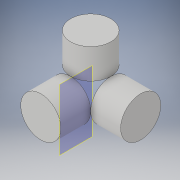
# Autodesk Inventor part: 3-way 90 1 Inch
Saved by Autodesk Inventor 2018 (Build 220112000, 112)
## iProperties
Created: 2018-01-18
Part Number: 3-way 90 1 Inch
Material: Generic
Document SubType Name: Modeling
Designer: owner
Density: 1 g/cm^3
Appearance: Default
Author: owner
Autodesk Inventor part; units mm, degrees
ref_plane "YZ Plane" through (0, 0, 0) normal (1, 0, 0) x (0, 1, 0)
ref_plane "XZ Plane" through (0, 0, 0) normal (0, 1, 0) x (-1, 0, 0)
ref_plane "XY Plane" through (0, 0, 0) normal (0, 0, 1) x (1, 0, 0)
sketch "Sketch11" plane through (0, 0, 0) normal (0, 0, 1) x (1, 0, 0)
  circle A0 centre (0, 0) radius 20.3835
  dimension "d30" = 40.767
  constraints: 1 centre point, 1 coincident
  measures "d30" diameter of A0
extrude "Extrusion7" add sketch "Sketch11" against normal blind 30.4292
sketch "Sketch12" plane through (0, 0, -30.4292) normal (0, 0, -1) x (-1, 0, 0)
  circle A0 centre (0, 0) radius 20.3835 projected
  line L0 (-20.3835, 0) -> (-20.3835, 36.5355)
  line L1 (0, 20.3835) -> (-34.8493, 20.3835)
  constraints: 4 end point, 2 point on circle, 2 tangent, 1 horizontal, 1 vertical
ref_plane "Work Plane4" through (20.3835, 0, -30.4292) normal (-1, 0, 0) x (0, 1, 0)
sketch "Sketch13" plane through (20.3835, 0, -30.4292) normal (-1, 0, 0) x (0, 1, 0)
  line L0 (0, -30.4292) -> (0, 20.3708)
  circle A0 centre (0, 20.3708) radius 20.3835
  line L1 (20.3835, 0) -> (-20.3835, 0) projected
  line L2 (0, 0) -> (51.1498, 0)
  line L3 (20.3835, -30.4292) -> (-20.3835, -30.4292) projected
  line L4 (5.5933, -30.4292) -> (5.5933, 0)
  line L5 (0, -0.0127) -> (0, -30.4292)
  dimension "d35" = 40.767
  dimension "d34" = 50.8
  constraints: 8 end point, 3 point on line, 2 collinear, 1 coincident, 1 midpoint, 1 perpendicular, 1 vertical, 1 vertical alignment, 2 other
  measures "d34" distance of L0.start L0.end
sketch "Sketch14" plane through (0, 0, 0) normal (0, 0, 1) x (1, 0, 0)
  line L0 (0, 0) -> (50.8, 0)
  line L1 (0, 0) -> (0, 50.8)
  dimension "d36" = 50.8
  dimension "d42" = 50.8
  constraints: 4 end point, 1 horizontal, 1 vertical
  measures "d36" distance of L0.start L0.end
  measures "d42" distance of L0.start L1.end
ref_plane "Work Plane5" through (50.8, 0, 0) normal (1, 0, 0) x (0, 1, 0)
extrude "Extrusion8" add sketch "Sketch13" against normal blind 30.4038 contours A0 L1 L0 | L0 L1 A0 | L1 A0
ref_plane "Work Plane6" through (0, 20.3835, -30.4292) normal (0, 1, 0) x (1, 0, 0)
sketch "Sketch15" plane through (0, 20.3835, -30.4292) normal (0, 1, 0) x (1, 0, 0)
  line L0 (0, -30.4292) -> (0, 20.3708)
  line L1 (0, 20.3708) -> (50.8, 20.3962)
  line L2 (50.8, 40.7797) -> (50.8, 0.0127) projected
  circle A0 centre (0, 20.3708) radius 20.3835
  dimension "d40" = 50.8
  dimension "d41" = 40.767
  constraints: 4 end point, 1 centre point, 1 coincident, 1 midpoint, 1 vertical
  measures "d40" distance of L0.start L0.end
  measures "d41" diameter of A0
ref_plane "Work Plane7" through (0, 50.8, 0) normal (0, 1, 0) x (-1, 0, 0)
extrude "Extrusion9" add sketch "Sketch15" along normal up to surface (30.4165 mm away)
sketch "Sketch16" plane through (0, 20.3835, -50.8) normal (0, -1, 0) x (0.7071068, 0, -0.7071068)
  circle A0 centre (-5.9702, 14.4133) radius 20.3835
  line L0 (14.4133, 14.4133) -> (-14.2542, 43.0808)
  line L1 (-21.5077, 50.3343) -> (0.009, 28.8176) projected
  line L2 (-28.8176, -0.009) -> (0.009, 28.8176) projected
  line L3 (-14.4043, 14.4043) -> (46.863, 14.4043)
  point P0 (-35.921, 35.921)
  constraints: 4 end point, 1 horizontal, 1 horizontal alignment, 1 midpoint, 1 point on line, 2 other
revolve "Revolution11" [suppressed]
revolve "Revolution7" [suppressed]
revolve "Revolution10" [suppressed]
body "Solid2"
